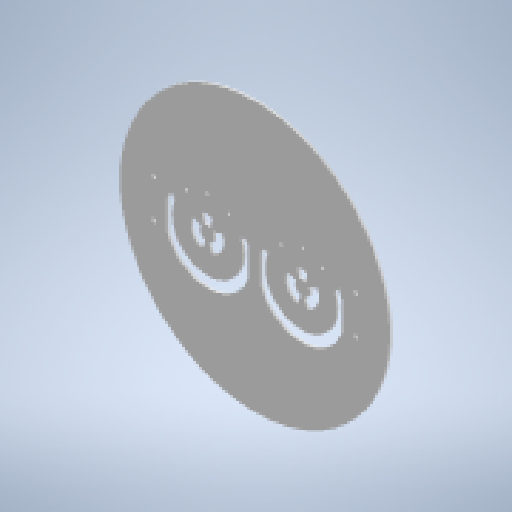
# Autodesk Inventor part: Деталь1
Saved by Autodesk Inventor 2023.2 (Build 272271030, 271C)
## iProperties
Created: 2024-01-26
Part Number: Деталь1
Material: Типовые
Document SubType Name: Modeling
Designer: I9232
Density: 1 g/cm^3
Appearance: По умолчанию
Author: I9232
Autodesk Inventor part; units mm, degrees
ref_plane "YZ Plane" through (0, 0, 0) normal (1, 0, 0) x (0, 1, 0)
ref_plane "XZ Plane" through (0, 0, 0) normal (0, 1, 0) x (-1, 0, 0)
ref_plane "XY Plane" through (0, 0, 0) normal (0, 0, 1) x (1, 0, 0)
sketch "Эскиз1" plane through (0, 0, 0) normal (0, 0, 1) x (1, 0, 0)
  circle A0 centre (-95.6307, 0) radius 127.844
  point P0 (0, 0)
  constraints: 1 centre point
extrude "Выдавливание1" add sketch "Эскиз1" along normal blind 2
sketch "Эскиз2" plane through (-95.6307, 0, 2) normal (0, 0, 1) x (1, 0, 0)
  circle A0 centre (-95.8398, -17.9366) radius 2 projected
  circle A1 centre (-95.8398, 17.9366) radius 2 projected
  circle A2 centre (95.6307, 17.9366) radius 2 projected
  circle A3 centre (95.6307, -17.9366) radius 2 projected
  circle A4 centre (64.7979, 22.6483) radius 1.5 projected
  circle A5 centre (45.3808, 29.2698) radius 1.5 projected
  circle A6 centre (24.6424, 22.2463) radius 1.5 projected
  circle A7 centre (-24.8516, 22.2463) radius 1.5 projected
  circle A8 centre (-45.59, 29.2698) radius 1.5 projected
  circle A9 centre (-65.0071, 22.6483) radius 1.5 projected
  arc A10 (82.9146, 5.6781) -> (79.467, 13.2351) centre (44.0811, -7.4733) ccw projected
  line L0 (79.467, 13.2351) -> (75.467, 8.6915) projected
  arc A11 (12.6952, 9.5242) -> (75.467, 8.6915) centre (43.9056, -4.1185) ccw projected
  line L1 (12.6952, 9.5242) -> (6.7704, 9.5242) projected
  arc A12 (6.7704, 9.5242) -> (5.2476, 5.6781) centre (44.0811, -7.4733) ccw projected
  line L2 (5.2476, 5.6781) -> (5.6979, -21.8861) projected
  arc A13 (5.6979, -21.8861) -> (82.4643, -21.8861) centre (44.0811, -7.4733) ccw projected
  line L3 (82.4643, -21.8861) -> (82.9146, 5.6781) projected
  line L4 (-83.7855, 5.6781) -> (-83.3353, -21.8861) projected
  arc A14 (-83.3353, -21.8861) -> (-6.5688, -21.8861) centre (-44.952, -7.4733) ccw projected
  line L5 (-6.5688, -21.8861) -> (-6.1185, 5.6781) projected
  arc A15 (-6.1185, 5.6781) -> (-7.6414, 9.5242) centre (-44.952, -7.4733) ccw projected
  line L6 (-7.6414, 9.5242) -> (-13.5662, 8.6915) projected
  arc A16 (-76.3379, 8.6915) -> (-13.5662, 8.6915) centre (-44.952, -4.1724) ccw projected
  line L7 (-76.3379, 8.6915) -> (-80.3379, 13.2351) projected
  arc A17 (-80.3379, 13.2351) -> (-83.7855, 5.6781) centre (-44.952, -7.4733) ccw projected
  arc A18 (49.9846, 10.9895) -> (40.0098, 11) centre (44.9818, -3.6809) ccw projected
  line L8 (40.0098, 11) -> (41.7858, 2.6976) projected
  arc A19 (48.1452, 2.8147) -> (41.7858, 2.6976) centre (45.0803, -3.4786) ccw projected
  line L9 (48.1452, 2.8147) -> (49.9846, 10.9895) projected
  line L10 (-41.995, 2.6976) -> (-40.2189, 11) projected
  arc A20 (-40.2189, 11) -> (-50.1937, 10.9895) centre (-45.191, -3.6809) ccw projected
  line L11 (-50.1937, 10.9895) -> (-48.3544, 2.8147) projected
  arc A21 (-41.995, 2.6976) -> (-48.3544, 2.8147) centre (-45.2895, -3.4786) ccw projected
  arc A22 (-40.2358, -18.3675) -> (-31.1913, 2.9719) centre (-45.191, -3.6809) ccw projected
  line L12 (-31.1913, 2.9719) -> (-39.3837, 0.2793) projected
  arc A23 (-43.2908, -10.1872) -> (-39.3837, 0.2793) centre (-45.2895, -3.4786) ccw projected
  line L13 (-43.2908, -10.1872) -> (-40.2358, -18.3675) projected
  arc A24 (30.9822, 2.9719) -> (40.0266, -18.3675) centre (44.9818, -3.6809) ccw projected
  line L14 (40.0266, -18.3675) -> (43.0816, -10.1872) projected
  arc A25 (39.1746, 0.2793) -> (43.0816, -10.1872) centre (45.0803, -3.4786) ccw projected
  line L15 (39.1746, 0.2793) -> (30.9822, 2.9719) projected
  arc A26 (49.9368, -18.3676) -> (58.9662, 3.0039) centre (44.9818, -3.6809) ccw projected
  line L16 (58.9662, 3.0039) -> (50.9531, 0.3306) projected
  arc A27 (46.9041, -10.2369) -> (50.9531, 0.3306) centre (45.0803, -3.4786) ccw projected
  line L17 (46.9041, -10.2369) -> (49.9368, -18.3676) projected
  arc A28 (-51.1623, 0.3306) -> (-47.1133, -10.2369) centre (-45.2895, -3.4786) ccw projected
  line L18 (-51.1623, 0.3306) -> (-59.1754, 3.0039) projected
  arc A29 (-59.1754, 3.0039) -> (-50.1459, -18.3676) centre (-45.191, -3.6809) ccw projected
  line L19 (-50.1459, -18.3676) -> (-47.1133, -10.2369) projected
  circle A30 centre (-54.8176, 7.1605) radius 0.675 projected
  circle A31 centre (-35.5643, 7.1605) radius 0.675 projected
  circle A32 centre (-45.191, -17.468) radius 0.675 projected
  circle A33 centre (54.6084, 7.1605) radius 0.675 projected
  circle A34 centre (44.9818, -17.468) radius 0.675 projected
  circle A35 centre (35.3552, 7.1605) radius 0.675 projected
  point P0 (95.6307, 0)
extrude "Выдавливание2" cut sketch "Эскиз2" against normal through all
sketch "Эскиз3" plane through (-95.6307, 0, 2) normal (0, 0, 1) x (1, 0, 0)
  circle A0 centre (0, 0) radius 127.844 projected
  line L0 (121.9057, 38.5109) -> (-121.9057, 38.5109)
  line L1 (121.35, 40.2278) -> (-121.35, 40.2278)
  arc A1 (-121.35, 40.2278) -> (-121.9057, 38.5109) centre (0, 0) ccw
  arc A2 (121.9057, 38.5109) -> (121.35, 40.2278) centre (0, 0) ccw
  point P0 (95.6307, 0)
  constraints: 8 point on circle, 4 end point, 2 centre point, 1 concentric, 1 horizontal, 1 parallel
extrude "Выдавливание3" cut sketch "Эскиз3" against normal blind 10 contours L0 A0 L1
